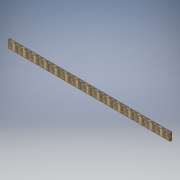
# Autodesk Inventor part: SideLong
Saved by Autodesk Inventor 2017 (Build 210142000, 142)
## iProperties
Created: 2016-10-24
Part Number: SideLong
Material: Generic
Document SubType Name: Modeling
Designer: andrew
Density: 1 g/cm^3
Appearance: Driftwood
d0: 80.000 in
Author: andrew
Autodesk Inventor part; units mm, degrees
ref_plane "YZ Plane" through (0, 0, 0) normal (1, 0, 0) x (0, 1, 0)
ref_plane "XZ Plane" through (0, 0, 0) normal (0, 1, 0) x (-1, 0, 0)
ref_plane "XY Plane" through (0, 0, 0) normal (0, 0, 1) x (1, 0, 0)
sketch "Sketch1" plane through (0, 0, 0) normal (0, 0, 1) x (1, 0, 0)
  line L0 (-1016, -50.8) -> (1016, -50.8)
  line L1 (1016, -50.8) -> (1016, 50.8)
  line L2 (1016, 50.8) -> (-1016, 50.8)
  line L3 (-1016, 50.8) -> (-1016, -50.8)
  line L4 (-1016, -50.8) -> (1016, 50.8) construction
  line L5 (1016, -50.8) -> (-1016, 50.8) construction
  point P0 (0, 0)
  dimension "d0" = 2032
  dimension "d1" = 101.6
  constraints: 12 end point, 2 midpoint, 2 parallel, 1 horizontal, 1 perpendicular
  measures "d0" distance of L1.end L2.end
  measures "d1" distance of L2.end L0.start
extrude "Extrusion1" add sketch "Sketch1" along normal blind 28.575
fillet "Fillet1" radius 9.525 4 edges at (0, 50.8, 0) (0, 50.8, 28.575) (0, -50.8, 0) (0, -50.8, 28.575)
body "Solid1"
